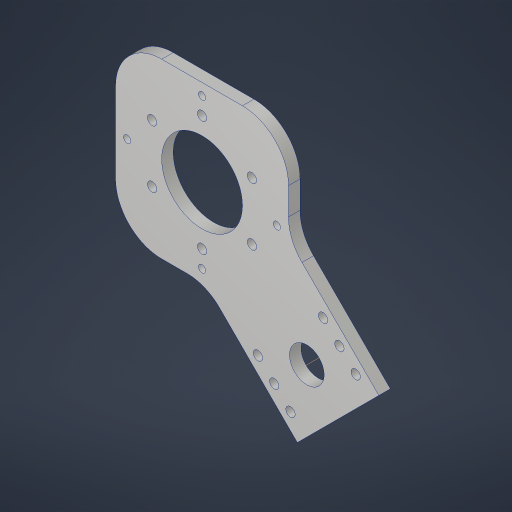
# Autodesk Inventor part: GP6-004
Saved by Autodesk Inventor 2023.4 (Build 274418000, 418)
## iProperties
RuleStatus: InUse
Created: 2025-02-23
Part Number: GP6-004
Material: Aluminum 6061
Document SubType Name: Modeling
Designer: brand
Mass: 132.735 g
Surface Area: 177.419 cm^2
Volume: 49.1612 cm^3
Density: 2.7 g/cm^3
Appearance: Aluminum - Flat
AfterDocNew0: SHOW
AfterDocOpen0: SHOW
Author: brand
Autodesk Inventor part; units mm, degrees
ref_plane "YZ Plane" through (0, 0, 0) normal (1, 0, 0) x (0, 1, 0)
ref_plane "XZ Plane" through (0, 0, 0) normal (0, 1, 0) x (-1, 0, 0)
ref_plane "XY Plane" through (0, 0, 0) normal (0, 0, 1) x (1, 0, 0)
sketch "Sketch1" plane through (0, 0, 0) normal (0, 0, 1) x (1, 0, 0)
  line L0 (-47.625, -47.625) -> (47.625, -47.625)
  line L1 (47.625, -47.625) -> (47.625, 47.625)
  line L2 (47.625, 47.625) -> (-47.625, 47.625)
  line L3 (-47.625, 47.625) -> (-47.625, -47.625)
  line L4 (-47.625, -47.625) -> (47.625, 47.625) construction
  line L5 (47.625, -47.625) -> (-47.625, 47.625) construction
  point P0 (0, 0)
  dimension "width" = 95.25
  dimension "length" = 95.25
  constraints: 12 end point, 2 midpoint, 2 parallel, 1 horizontal, 1 perpendicular
  measures "width" distance of L2.end L1.end
  measures "length" distance of L0.end L1.end
extrude "Extrusion1" add sketch "Sketch1" along normal mid plane 6.35
sketch "Sketch2" plane through (0, 0, 3.175) normal (0, 0, 1) x (1, 0, 0)
  circle A0 centre (0, 0) radius 35
  circle A1 centre (0, 0) radius 60 construction
  circle A2 centre (0, 0) radius 47.5
  line L0 (0, 35) -> (0, 60) construction
  line L1 (0, 47.5) -> (0, 35) construction
  point P0 (0, 41.25)
  point P1 (-41.25, 0)
  point P2 (0, -41.25)
  point P3 (41.25, 0)
  dimension "d4" = 70
  dimension "d5" = 120
  dimension "d8" = 360
  constraints: 4 end point, 4 vertical alignment, 3 coincident, 2 midpoint, 2 vertical, 11 other
hole "Hole1" at (0, 41.25, 3.175) at (-41.25, 0, 3.175) at (0, -41.25, 3.175) at (41.25, 0, 3.175) direction (0, 0, -1) diameter 3.9624 end through all thread size "10-32 UNF" class "2B" standard "ANSI Unified Screw Threads"
sketch "Sketch3" plane through (0, 0, 3.175) normal (0, 0, 1) x (1, 0, 0)
  circle A0 centre (0, 0) radius 31.75 construction
  point P0 (0, 31.75)
  point P1 (-27.4963, 15.875)
  point P2 (-27.4963, -15.875)
  point P3 (0, -31.75)
  point P4 (27.4963, -15.875)
  point P5 (27.4963, 15.875)
  dimension "d17" = 63.5
  dimension "d20" = 360
  constraints: 2 vertical alignment, 1 coincident, 9 other
hole "Hole2" at (0, 31.75, 3.175) at (-27.4963, 15.875, 3.175) at (-27.4963, -15.875, 3.175) at (0, -31.75, 3.175) at (27.4963, -15.875, 3.175) at (27.4963, 15.875, 3.175) direction (0, 0, -1) diameter 5.1054 end through all clearance for "Hex Machine Screw" size "#10" standard "Ansi Unified Screw Threads"
fillet "Fillet1" radius 25.4 1 edges at (-47.625, 47.625, 0)
sketch "Sketch4" plane through (0, 0, 3.175) normal (0, 0, 1) x (1, 0, 0)
  circle A0 centre (0, 0) radius 22.225
  dimension "d30" = 44.45
  constraints: 1 centre point, 1 coincident
  measures "d30" diameter of A0
extrude "Extrusion2" cut sketch "Sketch4" against normal through all
sketch "Sketch5" plane through (0, 0, 3.175) normal (0, 0, 1) x (1, 0, 0)
  circle A0 centre (0, 0) radius 64 construction
  circle A1 centre (57.721, -58.2433) radius 18 construction
  line L0 (95.821, 47.9105) -> (95.821, -47.9105) construction
  line L1 (66.7013, -31.3026) -> (30.7802, -67.2236) construction
  line L2 (30.7802, -67.2236) -> (39.7605, -76.2038) construction
  line L3 (48.7407, -49.2631) -> (57.721, -58.2433) construction
  line L4 (-47.625, -47.625) -> (47.625, -47.625) construction
  line L5 (2.2014, -47.625) -> (52.4884, -97.912)
  line L6 (52.4884, -97.912) -> (97.3897, -53.0107)
  line L7 (97.3897, -53.0107) -> (47.625, -3.2461)
  line L8 (47.625, -47.625) -> (47.625, 47.625) construction
  line L9 (2.2014, -47.625) -> (47.625, -47.625)
  line L10 (47.625, -47.625) -> (47.625, -3.2461)
  circle A2 centre (57.721, -58.2433) radius 9.525
  point P0 (95.821, 0)
  point P1 (39.7605, -76.2038)
  point P2 (48.7407, -85.1841)
  point P3 (75.6815, -40.2828)
  point P4 (75.6815, -40.2828)
  point P5 (84.6618, -49.2631)
  point P6 (-22.225, -47.625)
  dimension "d33" = 128
  dimension "d34" = 36
  dimension "d35" = 95.821
  dimension "d36" = 95.821
  dimension "d37" = 50.8
  dimension "d38" = 12.7
  dimension "d39" = 12.7
  dimension "d42" = 12.7
  dimension "d47" = 45
  dimension "d48" = 38.1
  dimension "d49" = 6.35
  dimension "d50" = 24.35
  dimension "d51" = 6.35
  dimension "d55" = 19.05
  dimension "d64" = 45
  constraints: 18 end point, 4 coincident, 4 perpendicular, 4 symmetric about line, 3 centre point, 2 midpoint, 2 point on line, 1 collinear, 1 horizontal alignment, 1 tangent, 1 vertical, 3 other
  measures "d33" diameter of A0
  measures "d34" diameter of A1
  measures "d35" distance from line of L0 point (0, 0)
  measures "d36" distance of L0.start L0.end
  measures "d37" distance of L1.start L1.end
  measures "d38" distance of L1.end L2.end
  measures "d39" distance of L3.start L3.end
  measures "d42" distance of point (30.78, -67.224) point (39.76, -76.204)
  measures "d47" angle of L0 L3
  measures "d48" distance from line of L0 A1.centre
  measures "d49" distance from line of L7 point (66.701, -31.303)
  measures "d50" distance from line of A1.centre L6
  measures "d51" distance from line of L5 point (39.76, -76.204)
  measures "d55" diameter of A2
  measures "d64" angle of L0 L7
extrude "Extrusion3" add sketch "Sketch5" against normal up to surface (6.35 mm away)
hole "Hole3" at (30.7802, -67.2236, 3.175) at (39.7605, -76.2038, 3.175) at (48.7407, -85.1841, 3.175) at (66.7013, -31.3026, 3.175) at (84.6618, -49.2631, 3.175) at (75.6815, -40.2828, 3.175) direction (0, 0, -1) diameter 5.1054 end through all clearance for "Hex Machine Screw" size "#10" standard "Ansi Unified Screw Threads"
fillet "Fillet2" radius 25.4 4 edges at (47.625, -3.2461, 0) (2.2014, -47.625, 0) (47.625, 47.625, 0) (-47.625, -47.625, 0)
equation "\"d36\" = d35"
equation "\"d39\" = d38"
equation "\"d42\" = d38"
equation "\"d50\" = 0.5 * d34 + d49"
equation "\"d51\" = d49"
equation "\"d64\" = d47"
equation "\"d63\" = d29"
equation "\"d29\" = 25.4"
body "Solid1"
